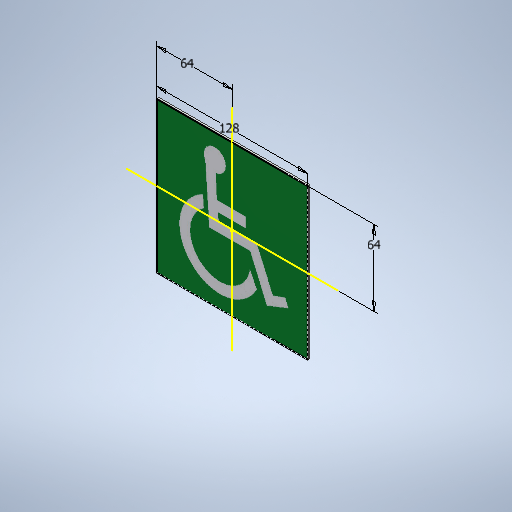
# Autodesk Inventor part: 장애인
Saved by Autodesk Inventor 2025.1 (Build 291241000, 241)
## iProperties
Created: 2024-10-28
Part Number: 장애인
Material: 일반
Document SubType Name: Modeling
Designer: gmsee
Density: 1 g/cm^3
Appearance: 기본값
Author: gmsee
Autodesk Inventor part; units mm, degrees
ref_plane "YZ Plane" through (0, 0, 0) normal (1, 0, 0) x (0, 1, 0)
ref_plane "XZ Plane" through (0, 0, 0) normal (0, 1, 0) x (-1, 0, 0)
ref_plane "XY Plane" through (0, 0, 0) normal (0, 0, 1) x (1, 0, 0)
sketch "스케치1" plane through (0, 0, 0) normal (0, 0, 1) x (1, 0, 0)
  line L0 (-64, 64) -> (64, 64) construction
  line L1 (64, 64) -> (64, -63.5224) construction
  line L2 (64, -63.5224) -> (-64, -63.5224) construction
  line L3 (-64, -63.5224) -> (-64, 64) construction
  line L4 (0, -89.0269) -> (0, 89.5045) projected
  line L5 (-89.6, 0) -> (89.6, 0) projected
  line L6 (-64, 64) -> (64, 64)
  line L7 (64, 64) -> (64, -63.5224)
  line L8 (64, -63.5224) -> (-64, -63.5224)
  line L9 (-64, -63.5224) -> (-64, 64)
  point P0 (0, 0)
  dimension "d1" = 128
  dimension "d9" = 64
  dimension "d10" = 64
  constraints: 8 end point, 2 parallel, 1 horizontal, 1 perpendicular, 2 other
  measures "d1" distance of L0.start L0.end
  measures "d9" distance between parallel lines of L4 L3
  measures "d10" distance between parallel lines of L0 L5
extrude "돌출1" add sketch "스케치1" against normal blind 2
